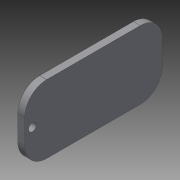
# Autodesk Inventor part: clamp
Saved by Autodesk Inventor 2015 SP1 (Build 190203100, 203)
## iProperties
Created: 2016-07-12
Part Number: clamp
Material: Generic
Document SubType Name: Modeling
Designer: lustinga
Density: 1 g/cm^3
Appearance: Default
Author: lustinga
Autodesk Inventor part; units mm, degrees
ref_plane "YZ Plane" through (0, 0, 0) normal (1, 0, 0) x (0, 1, 0)
ref_plane "XZ Plane" through (0, 0, 0) normal (0, 1, 0) x (-1, 0, 0)
ref_plane "XY Plane" through (0, 0, 0) normal (0, 0, 1) x (1, 0, 0)
sketch "Sketch1" plane through (0, 0, 0) normal (1, 0, 0) x (0, 1, 0)
  arc A0 (-27.0381, 32.6694) -> (2.4619, 32.6694) centre (-12.2881, 32.6694) ccw
  arc A1 (-27.0381, 32.6694) -> (2.4619, 32.6694) centre (-12.2881, 32.6694) ccw
  arc A2 (-27.0381, 32.6694) -> (2.4619, 32.6694) centre (-12.2881, 32.6694) ccw
  line L0 (-27.0381, 32.6694) -> (-27.0381, 50.6694)
  line L1 (2.4619, 32.6694) -> (2.4619, 50.6694)
  line L2 (-27.0381, 50.6694) -> (-37.7302, 50.6694)
  arc A3 (2.4619, 68.6694) -> (-27.0381, 68.6694) centre (-12.2881, 68.6694) ccw
  arc A4 (2.4619, 68.6694) -> (-27.0381, 68.6694) centre (-12.2881, 68.6694) ccw
  arc A5 (2.4619, 68.6694) -> (-27.0381, 68.6694) centre (-12.2881, 68.6694) ccw
  line L3 (-27.0381, 68.6694) -> (-27.0381, 50.6694)
  line L4 (2.4619, 68.6694) -> (2.4619, 50.6694)
  circle A6 centre (-12.2881, 22.6694) radius 1.875
  circle A7 centre (-12.2881, 78.6694) radius 1.875
  point P0 (0, 0)
  dimension "d7" = 29.5
  dimension "d8" = 29.5
  dimension "d9" = 29.5
  dimension "d12" = 18
  dimension "d13" = 18
  dimension "d14" = 3.75
  dimension "d16" = 3.75
  dimension "d17" = 56
  constraints: 12 point on circle, 10 end point, 9 symmetric about line, 8 centre point, 2 vertical, 1 horizontal, 3 other
  measures "d7" diameter of A0
  measures "d8" diameter of A1
  measures "d9" diameter of A2
  measures "d12" distance of L0.start L0.end
  measures "d13" distance of L1.start L1.end
  measures "d14" diameter of A6
  measures "d16" diameter of A7
  measures "d17" distance of A6.centre A7.centre
extrude "Extrusion1" add sketch "Sketch1" along normal blind 3.175
body "Solid1"
